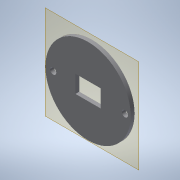
# Autodesk Inventor part: led_deckel
Saved by Autodesk Inventor 2020.2 (Build 242310000, 310)
## iProperties
Created: 2020-11-08
Part Number: led_deckel
Material: Generisch
Document SubType Name: Modeling
Designer: g.schardt
Density: 1 g/cm^3
Appearance: Vorgabe
Author: g.schardt
Autodesk Inventor part; units mm, degrees
ref_plane "YZ Plane" through (0, 0, 0) normal (1, 0, 0) x (0, 1, 0)
ref_plane "XZ Plane" through (0, 0, 0) normal (0, 1, 0) x (-1, 0, 0)
ref_plane "XY Plane" through (0, 0, 0) normal (0, 0, 1) x (1, 0, 0)
ref_plane "Arbeitsebene1" through (0, 0, 0) normal (0, 0, 1) x (1, 0, 0)
sketch "Skizze1" plane through (0, 0, 0) normal (0, 0, 1) x (1, 0, 0)
  circle A0 centre (0, 0) radius 22 projected
  point P0 (0, 0)
extrude "Extrusion1" add sketch "Skizze1" along normal blind 2
sketch "Skizze2" plane through (0, 0, 2) normal (0, 0, 1) x (1, 0, 0)
  circle A0 centre (-18, 0) radius 1.6 projected
  circle A1 centre (18, 0) radius 1.6 projected
  point P0 (0, 0)
  point P1 (19.0059, -0.5696)
hole "Bohrung1" at (-18, 0, 2) at (19.0059, -0.5696, 2) direction (0, 0, -1) diameter 3.2 end through all
sketch "Skizze3" plane through (0, 0, 2) normal (0, 0, 1) x (1, 0, 0)
  line L0 (6.5, -4.5) -> (-6.5, -4.5)
  line L1 (-6.5, -4.5) -> (-6.5, 4.5)
  line L2 (-6.5, 4.5) -> (6.5, 4.5)
  line L3 (6.5, 4.5) -> (6.5, -4.5)
  line L4 (6.5, -4.5) -> (-6.5, 4.5) construction
  line L5 (-6.5, -4.5) -> (6.5, 4.5) construction
  point P0 (0, 0)
  dimension "d9" = 13
  dimension "d10" = 9
  constraints: 12 end point, 2 midpoint, 2 parallel, 1 horizontal, 1 perpendicular
  measures "d9" distance of L1.end L2.end
  measures "d10" distance of L0.end L1.end
extrude "Extrusion2" cut sketch "Skizze3" against normal blind 10
